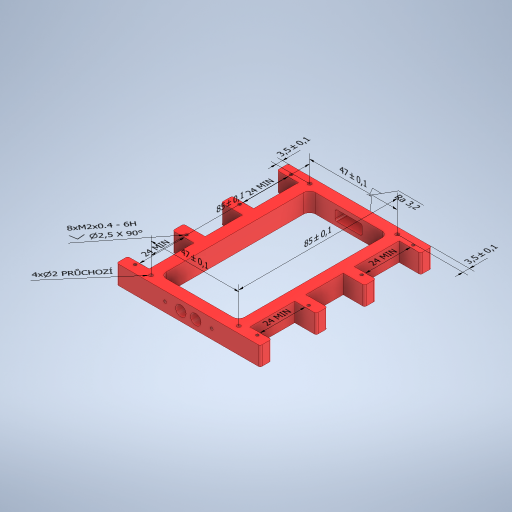
# Autodesk Inventor part: rapoukBasev5
Saved by Autodesk Inventor 2024 (Build 280153000, 153)
## iProperties
Created: 2024-01-02
Part Number: rapoukBasev5
Material: EN AW-6060 T6
Document SubType Name: Modeling
Designer: Roman Suk
Density: 2.7 g/cm^3
Appearance: Light Red
MASSSFP: 400 g
SFP: 4HR
Author: Roman Suk
Autodesk Inventor part; units mm, degrees
ref_plane "YZ Plane" through (0, 0, 0) normal (1, 0, 0) x (0, 1, 0)
ref_plane "XZ Plane" through (0, 0, 0) normal (0, 1, 0) x (-1, 0, 0)
ref_plane "XY Plane" through (0, 0, 0) normal (0, 0, 1) x (1, 0, 0)
sketch "Sketch2" plane through (0, 0, 0) normal (0, 1, 0) x (-1, 0, 0)
  line L0 (0, 0) -> (0, 40)
  line L1 (0, 40) -> (17.825, 40)
  line L2 (0, 40) -> (0, 46) construction
  line L3 (0, 46) -> (37.5, 46)
  line L4 (21, 36.825) -> (21, 0)
  line L5 (38.5, 45) -> (38.5, 41)
  line L6 (37.5, 40) -> (27, 40)
  line L7 (27, 40) -> (27, 16)
  line L8 (27, 16) -> (37.5, 16)
  line L9 (38.5, 15) -> (38.5, 11)
  line L10 (37.5, 10) -> (27, 10)
  line L11 (27, 10) -> (27, 0)
  line L12 (0, 0) -> (21, 0)
  line L13 (27, 28) -> (38.5, 28)
  arc A0 (21, 36.825) -> (17.825, 40) centre (17.825, 36.825) ccw
  arc A1 (38.5, 45) -> (37.5, 46) centre (37.5, 45) ccw
  arc A2 (37.5, 40) -> (38.5, 41) centre (37.5, 41) ccw
  arc A3 (38.5, 15) -> (37.5, 16) centre (37.5, 15) ccw
  arc A4 (37.5, 10) -> (38.5, 11) centre (37.5, 11) ccw
  line L14 (0, -40) -> (17.825, -40)
  line L15 (0, -46) -> (37.5, -46)
  line L16 (21, -36.825) -> (21, 0)
  line L17 (38.5, -45) -> (38.5, -41)
  line L18 (37.5, -40) -> (27, -40)
  line L19 (27, -40) -> (27, -16)
  line L20 (27, -16) -> (37.5, -16)
  line L21 (38.5, -15) -> (38.5, -11)
  line L22 (37.5, -10) -> (27, -10)
  line L23 (27, -10) -> (27, 0)
  arc A5 (17.825, -40) -> (21, -36.825) centre (17.825, -36.825) ccw
  arc A6 (37.5, -46) -> (38.5, -45) centre (37.5, -45) ccw
  arc A7 (38.5, -41) -> (37.5, -40) centre (37.5, -41) ccw
  arc A8 (37.5, -16) -> (38.5, -15) centre (37.5, -15) ccw
  arc A9 (38.5, -11) -> (37.5, -10) centre (37.5, -11) ccw
  line L24 (0, 40) -> (-17.825, 40)
  line L25 (0, 46) -> (-37.5, 46)
  line L26 (-21, 36.825) -> (-21, 0)
  line L27 (-38.5, 45) -> (-38.5, 41)
  line L28 (-37.5, 40) -> (-27, 40)
  line L29 (-27, 40) -> (-27, 16)
  line L30 (-27, 16) -> (-37.5, 16)
  line L31 (-38.5, 15) -> (-38.5, 11)
  line L32 (-37.5, 10) -> (-27, 10)
  line L33 (-27, 10) -> (-27, 0)
  arc A10 (-17.825, 40) -> (-21, 36.825) centre (-17.825, 36.825) ccw
  arc A11 (-37.5, 46) -> (-38.5, 45) centre (-37.5, 45) ccw
  arc A12 (-38.5, 41) -> (-37.5, 40) centre (-37.5, 41) ccw
  arc A13 (-37.5, 16) -> (-38.5, 15) centre (-37.5, 15) ccw
  arc A14 (-38.5, 11) -> (-37.5, 10) centre (-37.5, 11) ccw
  line L34 (0, -46) -> (-37.5, -46)
  arc A15 (-38.5, -45) -> (-37.5, -46) centre (-37.5, -45) ccw
  line L35 (-38.5, -45) -> (-38.5, -41)
  arc A16 (-37.5, -40) -> (-38.5, -41) centre (-37.5, -41) ccw
  line L36 (-37.5, -40) -> (-27, -40)
  line L37 (-27, -40) -> (-27, -16)
  line L38 (-27, -16) -> (-37.5, -16)
  arc A17 (-38.5, -15) -> (-37.5, -16) centre (-37.5, -15) ccw
  line L39 (-38.5, -15) -> (-38.5, -11)
  arc A18 (-37.5, -10) -> (-38.5, -11) centre (-37.5, -11) ccw
  line L40 (-37.5, -10) -> (-27, -10)
  line L41 (-27, -10) -> (-27, 0)
  line L42 (-21, -36.825) -> (-21, 0)
  line L43 (0, -40) -> (-17.825, -40)
  arc A19 (-21, -36.825) -> (-17.825, -40) centre (-17.825, -36.825) ccw
  line L44 (23.5, 42.5) -> (23.5, -46) construction
  point P0 (21, 40)
  point P1 (38.5, 46)
  point P2 (38.5, 40)
  point P3 (38.5, 16)
  point P4 (38.5, 10)
  point P5 (32.74, 41.8)
  point P6 (32.74, 14.2)
  point P7 (32.74, -41.8)
  point P8 (32.74, -14.2)
  point P9 (-32.74, 41.8)
  point P10 (-32.74, 14.2)
  point P11 (-32.74, -41.8)
  point P12 (-32.74, -14.2)
  point P13 (-23.5, 42.5)
  point P14 (23.5, -42.5)
  point P15 (-23.5, 42.5)
  point P16 (-23.5, -42.5)
  dimension "d2" = 40
  dimension "d3" = 6
  dimension "d4" = 38.5
  dimension "d5" = 21
  dimension "d6" = 6
  dimension "d7" = 11.5
  dimension "d8" = 24
  dimension "d9" = 11.5
  dimension "d10" = 6
  dimension "d11" = 11.5
  dimension "d12" = 5.74
  dimension "d13" = 27.6
  dimension "d14" = 3.175
  dimension "d15" = 1
  dimension "d37" = 47
  dimension "d174" = 85
  dimension "d176" = 92
  dimension "d177" = 3.5
  constraints: 90 end point, 68 symmetric about line, 40 point on circle, 20 centre point, 16 point on line, 10 tangent, 5 perpendicular, 5 vertical, 4 horizontal, 3 equal radius, 1 midpoint, 15 other
  measures "d2" distance of L0.start L0.end
  measures "d3" distance of L0.end L2.end
  measures "d4" distance of L2.end point (38.5, 46)
  measures "d5" distance of L0.end point (21, 40)
  measures "d6" distance of point (38.5, 46) point (38.5, 40)
  measures "d7" distance of point (38.5, 40) L6.end
  measures "d8" distance of L6.end L7.end
  measures "d9" distance of L7.end point (38.5, 16)
  measures "d10" distance of point (38.5, 16) point (38.5, 10)
  measures "d11" distance of point (38.5, 10) L10.end
  measures "d12" distance from line of point (32.74, 41.8) L7
  measures "d13" diameter of point (32.74, 41.8) L13
  measures "d14" radius of A0
  measures "d15" radius of A1
  measures "d37" diameter of L44.start L0
  measures "d174" distance of L44.start point (23.5, -42.5)
  measures "d176" distance between parallel lines of L25 L34
  measures "d177" distance from line of L15 point (23.5, -42.5)
extrude "Extrusion2" add sketch "Sketch2" along normal blind 10
hole "Hole1" at (-32.74, 0, 41.8) at (-32.74, 0, 14.2) at (-32.74, 0, -41.8) at (-32.74, 0, -14.2) at (32.74, 0, 41.8) at (32.74, 0, 14.2) at (32.74, 0, -14.2) at (32.74, 0, -41.8) direction (0, 1, 0) diameter 1.567 end through all countersink diameter 2.5 countersink angle 90 thread size "M2x0.4" class "6H" standard "ISO Metric profile"
hole "Hole2" at (-23.5, 0, 42.5) at (23.5, 0, 42.5) at (-23.5, 0, -42.5) at (23.5, 0, -42.5) direction (0, 1, 0) diameter 2 end through all
sketch "Sketch4" plane through (-37.5, 0, 46) normal (0, 0, 1) x (1, 0, 0)
  line L0 (37.5, 0) -> (37.5, 10) construction
  line L1 (0, 10) -> (75, 10) projected
  line L2 (-1, 0) -> (-1, 10) projected
  line L3 (-1, 5) -> (75, 5)
  circle A0 centre (41.5, 5) radius 2.8
  circle A1 centre (33.5, 5) radius 2.8
  point P0 (37.5, 5)
  point P1 (25, 5)
  point P2 (50, 5)
  dimension "d149" = 5.6
  dimension "d153" = 5.6
  dimension "d156" = 8
  dimension "d157" = 4
  dimension "d160" = 25
  dimension "d161" = 12.5
  constraints: 4 end point, 4 point on line, 3 midpoint, 2 centre point, 1 horizontal
  measures "d149" diameter of A0
  measures "d153" diameter of A1
  measures "d156" distance of A0.centre A1.centre
  measures "d157" distance from line of L0 A0.centre
  measures "d160" distance of point (50, 5) point (25, 5)
  measures "d161" distance from line of L0 point (50, 5)
extrude "Extrusion3" cut sketch "Sketch4" against normal up to surface (6 mm away)
hole "Hole3" at (-12.5, 5, 46) at (12.5, 5, 46) direction (0, 0, -1) diameter 1.567 depth 6.3 tip angle 118 thread size "M2x0.4" class "6H" standard "ISO Metric profile"
sketch "Sketch6" plane through (37.5, 0, -46) normal (0, 0, -1) x (-1, 0, 0)
  line L0 (0, 0) -> (0, 10) projected
  line L1 (0, 5) -> (75, 5)
  line L2 (75, 0) -> (75, 10) projected
  line L3 (37.5, 0) -> (37.5, 10) construction
  line L4 (31.25, 2.25) -> (43.75, 2.25)
  line L5 (44.75, 3.25) -> (44.75, 6.75)
  line L6 (43.75, 7.75) -> (31.25, 7.75)
  line L7 (30.25, 6.75) -> (30.25, 3.25)
  line L8 (30.25, 2.25) -> (44.75, 7.75) construction
  line L9 (44.75, 2.25) -> (30.25, 7.75) construction
  line L10 (0, 10) -> (75, 10) projected
  line L11 (75, 0) -> (75, 10) projected
  arc A0 (43.75, 2.25) -> (44.75, 3.25) centre (43.75, 3.25) ccw
  arc A1 (30.25, 3.25) -> (31.25, 2.25) centre (31.25, 3.25) ccw
  arc A2 (31.25, 7.75) -> (30.25, 6.75) centre (31.25, 6.75) ccw
  arc A3 (44.75, 6.75) -> (43.75, 7.75) centre (43.75, 6.75) ccw
  point P0 (37.5, 5)
  point P1 (37.5, 5)
  dimension "d169" = 14.5
  dimension "d170" = 5.5
  dimension "d173" = 1
  constraints: 16 end point, 8 midpoint, 8 point on circle, 8 point on line, 8 tangent, 4 centre point, 3 equal radius, 2 parallel, 1 horizontal, 1 horizontal alignment, 1 perpendicular, 1 vertical, 1 vertical alignment
  measures "d169" distance of L9.end L8.end
  measures "d170" distance of L8.end L9.start
  measures "d173" radius of A0
extrude "Extrusion4" cut sketch "Sketch6" against normal up to surface (6 mm away) contours L7 A2 L6 A3 L5 L1 | L1 L5 A0 L4 A1 L7
equation "\"d6\" = d3"
equation "\"d9\" = d7"
equation "\"d10\" = d3"
equation "\"d11\" = d7"
body "Solid2"
